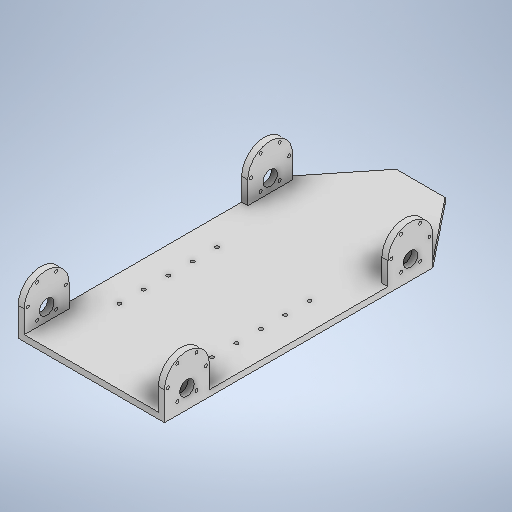
# Autodesk Inventor part: Base
Saved by Autodesk Inventor 2025 (Build 290162010, 162A)
## iProperties
Created: 2024-09-12
Part Number: Base
Material: Generic
Document SubType Name: Modeling
Designer: fist5
Density: 1 g/cm^3
Appearance: Default
Author: fist5
Autodesk Inventor part; units mm, degrees
ref_plane "YZ Plane" through (0, 0, 0) normal (1, 0, 0) x (0, 1, 0)
ref_plane "XZ Plane" through (0, 0, 0) normal (0, 1, 0) x (-1, 0, 0)
ref_plane "XY Plane" through (0, 0, 0) normal (0, 0, 1) x (1, 0, 0)
sketch "Sketch1" plane through (0, 0, 0) normal (0, 1, 0) x (-1, 0, 0)
  line L0 (60, 135) -> (-60, 135)
  line L1 (-60, 135) -> (-60, -135)
  line L2 (-60, -135) -> (60, -135)
  line L3 (60, -135) -> (60, 135)
  line L4 (60, 135) -> (-60, -135) construction
  line L5 (-60, 135) -> (60, -135) construction
  point P0 (0, 0)
  dimension "d0" = 270
  dimension "d1" = 120
  constraints: 12 end point, 2 midpoint, 2 parallel, 1 horizontal, 1 perpendicular
  measures "d0" distance between parallel lines of L0 L2
  measures "d1" distance between parallel lines of L1 L3
extrude "Extrusion1" add sketch "Sketch1" along normal blind 5
sketch "Sketch2" plane through (0, 5, 0) normal (0, 1, 0) x (1, 0, 0)
  line L0 (60, 135) -> (-60, 135) projected
  line L1 (20, 135) -> (60, 85)
  line L2 (60, -135) -> (60, 135) projected
  line L3 (-20, 135) -> (-60, 85)
  line L4 (-60, 135) -> (-60, -135) projected
  line L5 (60, 85) -> (60, 135)
  line L6 (-20, 135) -> (-60, 135)
  point P0 (0, 0)
  point P1 (-60, 0)
  point P2 (60, 0)
  point P3 (-20, 135)
  point P4 (0, 135)
  dimension "d5" = 40
  dimension "d6" = 50
  dimension "d7" = 50
  dimension "d38" = 20
  constraints: 8 end point, 3 midpoint, 3 point on line, 3 vertical alignment, 2 collinear, 2 horizontal alignment
  measures "d5" distance of L3.start L1.start
  measures "d6" distance of L0.start L1.end
  measures "d7" vertical distance of L3.end L3.start
  measures "d38" distance of L1.start point (0, 135)
extrude "Extrusion2" cut sketch "Sketch2" against normal up to next
sketch "Sketch3" plane through (-60, 0, 135) normal (-1, 0, 0) x (0, 0, 1)
  line L0 (-220, 5) -> (0, 5) projected
  line L1 (-220, 0) -> (0, 0) projected
  line L2 (-220, 5) -> (-220, 0) projected
  line L3 (0, 0) -> (0, 5) projected
  circle A0 centre (-201.62, 23.38) radius 18.38
  circle A1 centre (-18.38, 23.38) radius 18.38
  line L4 (-220, 23.38) -> (-220, 2.5)
  line L5 (-36.76, 23.38) -> (-36.76, 0)
  line L6 (0, 23.38) -> (0, 1.3847)
  line L7 (-183.24, 23.38) -> (-183.24, 0)
  point P0 (-135, 0)
  point P1 (0, 2.5)
  point P2 (0, 2.5)
  point P3 (-36.76, 5)
  point P4 (-183.24, 5)
  dimension "d11" = 36.76
  dimension "d12" = 36.76
  dimension "d13" = 18.38
  dimension "d15" = 18.38
  constraints: 8 end point, 6 tangent, 4 point on circle, 3 midpoint, 3 point on line, 2 centre point, 2 perpendicular
  measures "d11" diameter of A0
  measures "d12" diameter of A1
  measures "d13" horizontal distance of L4.end A0.centre
  measures "d15" horizontal distance of point (0, 2.5) A1.centre
extrude "Extrusion3" add sketch "Sketch3" against normal blind 5 contours L4 A0 L0 | A0 L7 L0 | A0 | L5 A1 L0 | A1 L6 L0 | A1
sketch "Sketch4" plane through (60, 0, 135) normal (1, 0, 0) x (0, 0, -1)
  line L0 (36.76, 5) -> (36.76, 23.38) projected
  arc A0 (36.76, 23.38) -> (0, 23.38) centre (18.38, 23.38) ccw projected
  line L1 (0, 23.38) -> (0, 5) projected
  line L2 (36.76, 5) -> (0, 5) projected
  line L3 (220, 5) -> (220, 23.38) projected
  arc A1 (220, 23.38) -> (183.24, 23.38) centre (201.62, 23.38) ccw projected
  line L4 (183.24, 23.38) -> (183.24, 5) projected
  line L5 (220, 5) -> (183.24, 5) projected
  point P0 (135, 0)
extrude "Extrusion4" add sketch "Sketch4" against normal blind 5
sketch "Sketch5" plane through (-60, 0, -85) normal (-1, 0, 0) x (0, 0, 1)
  circle A0 centre (18.38, 15.48) radius 5.98
  circle A1 centre (201.62, 15.48) radius 5.98
  arc A2 (36.76, 23.38) -> (0, 23.38) centre (18.38, 23.38) ccw projected
  arc A3 (220, 23.38) -> (183.24, 23.38) centre (201.62, 23.38) ccw projected
  circle A4 centre (18.38, 23.38) radius 15.605
  circle A5 centre (2.775, 23.38) radius 1.255
  circle A6 centre (10.5775, 9.8657) radius 1.255
  circle A7 centre (26.1825, 9.8657) radius 1.255
  circle A8 centre (33.985, 23.38) radius 1.255
  circle A9 centre (26.1825, 36.8943) radius 1.255
  circle A10 centre (10.5775, 36.8943) radius 1.255
  circle A11 centre (201.62, 23.38) radius 15.605
  circle A12 centre (186.015, 23.38) radius 1.255
  circle A13 centre (193.8175, 9.8657) radius 1.255
  circle A14 centre (209.4225, 9.8657) radius 1.255
  circle A15 centre (217.225, 23.38) radius 1.255
  circle A16 centre (209.4225, 36.8943) radius 1.255
  circle A17 centre (193.8175, 36.8943) radius 1.255
  point P0 (85, 0)
  dimension "d26" = 31.21
  dimension "d32" = 31.21
  dimension "d20" = 11.96
  dimension "d21" = 11.96
  dimension "d22" = 7.9
  dimension "d23" = 7.9
  dimension "d27" = 2.51
  dimension "d30" = 360
  dimension "d33" = 2.51
  dimension "d36" = 360
  constraints: 14 centre point, 4 horizontal alignment, 2 coincident, 2 vertical alignment, 30 other
  measures "d20" diameter of A1
  measures "d21" diameter of A0
  measures "d22" distance of A0.centre A2.centre
  measures "d23" distance of A1.centre A3.centre
  measures "d27" diameter of A5
  measures "d33" diameter of A12
extrude "Extrusion5" cut sketch "Sketch5" against normal up to surface (120 mm away) contours A0 | A1 | A4 A8 | A4 A8 | A9 A4 | A4 A9 | A7 A4 | A4 A7 | A10 A4 | A4 A10 | A6 A4 | A4 A6 | A5 A4 | A4 A5 | A11 A15 | A11 A15 | A16 A11 | A11 A16 | A14 A11 | A11 A14 | A17 A11 | A11 A17 | A13 A11 | A11 A13 | A12 A11 | A11 A12
sketch "Sketch6" plane through (0, 5, 0) normal (0, 1, 0) x (1, 0, 0)
  line L0 (60, -98.24) -> (55, -98.24) projected
  line L1 (-38, 6) -> (-38, -74)
  line L2 (-38, -74) -> (38, -74)
  line L3 (38, -74) -> (38, 6)
  line L4 (38, 6) -> (-38, 6)
  line L5 (-38, 6) -> (38, -74) construction
  line L6 (-38, -74) -> (38, 6) construction
  circle A0 centre (38, 6) radius 1.5
  circle A1 centre (38, -14) radius 1.5
  circle A2 centre (38, -34) radius 1.5
  circle A3 centre (38, -54) radius 1.5
  circle A4 centre (38, -74) radius 1.5
  circle A5 centre (-38, 6) radius 1.5
  circle A6 centre (-38, -14) radius 1.5
  circle A7 centre (-38, -34) radius 1.5
  circle A8 centre (-38, -54) radius 1.5
  circle A9 centre (-38, -74) radius 1.5
  point P0 (0, 0)
  point P1 (0, -34)
  point P2 (57.5, -98.24)
  dimension "d39" = 64.24
  dimension "d40" = 76
  dimension "d41" = 80
  dimension "d42" = 3
  dimension "d45" = 20
  dimension "d48" = 76
  constraints: 12 end point, 10 centre point, 3 midpoint, 2 parallel, 2 vertical, 1 coincident, 1 horizontal, 1 perpendicular, 1 vertical alignment, 18 other
  measures "d39" vertical distance of point (57.5, -98.24) point (0, -34)
  measures "d40" distance between parallel lines of L1 L3
  measures "d41" distance between parallel lines of L4 L2
  measures "d42" diameter of A0
  measures "d45" distance of A0.centre A1.centre
  measures "d48" distance of A0.centre A5.centre
extrude "Extrusion6" cut sketch "Sketch6" against normal up to surface (5 mm away) contours L4 A5 L1 | L1 A5 L4 | A6 L1 | L1 A6 | A0 L3 L4 | L4 L3 A0 | A7 L1 | L1 A7 | A1 L3 | L3 A1 | A8 L1 | L1 A8 | A2 L3 | L3 A2 | A9 L2 L1 | L1 L2 A9 | A3 L3 | L3 A3 | A4 L3 L2 | L2 L3 A4
body "Solid1"
